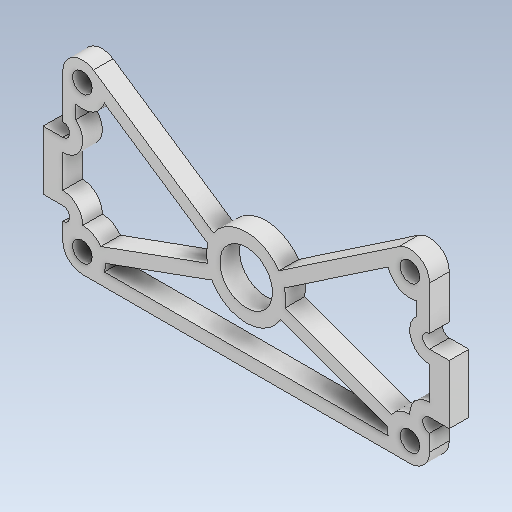
# Autodesk Inventor part: 横回転フレーム改３
Saved by Autodesk Inventor 2020 (Build 240168000, 168)
## iProperties
Created: 2020-02-25
Part Number: 横回転フレーム改３
Material: アルミニウム 2014-T4
Document SubType Name: Modeling
Designer: tanjihayato
Density: 2.8 g/cm^3
Appearance: サテン
Mass: 4.28179 g
Surface Area: 24.5942 cm^2
Volume: 1.52921 cm^3
Author: tanjihayato
Autodesk Inventor part; units mm, degrees
ref_plane "YZ Plane" through (0, 0, 0) normal (1, 0, 0) x (0, 1, 0)
ref_plane "XZ Plane" through (0, 0, 0) normal (0, 1, 0) x (-1, 0, 0)
ref_plane "XY Plane" through (0, 0, 0) normal (0, 0, 1) x (1, 0, 0)
sketch "スケッチ1" plane through (0, 0, 0) normal (0, 0, 1) x (1, 0, 0)
  line L0 (0, 0) -> (0, 4) construction
  line L1 (0, 0) -> (8.6476, -12.2564)
  line L2 (8.6476, -12.2564) -> (-0.2755, 4.5179)
  circle A0 centre (3.0119, -1.6621) radius 4
  line L3 (-57.3278, -140) -> (69.8706, -140)
  line L4 (3.0119, -1.6621) -> (117.7837, 59.3906)
  circle A1 centre (0, 0) radius 23.1
  circle A2 centre (0, -29.1039) radius 6.0039
  line L5 (0, 0) -> (0, -29.1039) construction
  circle A3 centre (0, -29.1039) radius 16.55
  circle A4 centre (0, -7.5039) radius 5.05
  circle A5 centre (0, 4) radius 3
  circle A6 centre (0, -7.5039) radius 20.05
  circle A7 centre (-14, 10.2376) radius 2.55
  circle A8 centre (14, 10.2376) radius 2.55
  circle A9 centre (14, -25.2454) radius 2.55
  circle A10 centre (-14, -25.2454) radius 2.55
  circle A11 centre (-14, 10.2376) radius 14
  circle A12 centre (14, 10.2376) radius 14
  circle A13 centre (14, -25.2454) radius 14
  circle A14 centre (-14, -25.2454) radius 14
  line L6 (-14, 10.2376) -> (-14, -25.2454) construction
  line L7 (-14, -25.2454) -> (14, -25.2454) construction
  circle A15 centre (0, 0) radius 9
  line L8 (-0.2755, 4.5179) -> (3.4816, -2.5449) construction
  line L9 (-2.9462, 3.0973) -> (0.8109, -3.9656)
  line L10 (6.1522, -1.1243) -> (2.3951, 5.9386)
  arc A16 (2.3951, 5.9386) -> (-2.9462, 3.0973) centre (-0.2755, 4.5179) ccw
  arc A17 (0.8109, -3.9656) -> (6.1522, -1.1243) centre (3.4816, -2.5449) ccw
  line L11 (-5, 2.8868) -> (5, 2.8868) construction
  line L12 (5, 2.8868) -> (0, -5.7735) construction
  line L13 (0, -5.7735) -> (-5, 2.8868) construction
  circle A18 centre (-5, 2.8868) radius 1.5
  circle A19 centre (5, 2.8868) radius 1.5
  circle A20 centre (0, -5.7735) radius 1.5
  line L14 (-28, 22.5965) -> (-28, -43.3295)
  line L15 (28, 22.9271) -> (28, -43.0008)
  line L16 (-28, 26.1991) -> (28, 26.1991)
  circle A21 centre (0, 0) radius 25.1
  line L17 (-28, -18.848) -> (28, -18.848)
  circle A22 centre (0, -29.1039) radius 8.0039
  circle A23 centre (-25, 23.1991) radius 3
  circle A24 centre (25, 23.1991) radius 3
  circle A25 centre (25, -38.2069) radius 3
  circle A26 centre (-25, -38.2069) radius 3
  circle A27 centre (-25, -15.848) radius 3
  circle A28 centre (25, -15.848) radius 3
  circle A29 centre (-25, -15.848) radius 4.5
  circle A30 centre (25, -15.848) radius 4.5
  circle A31 centre (0, -7.5039) radius 4.5
  circle A32 centre (0, -29.1039) radius 17.55
  circle A33 centre (0, -7.5039) radius 6.05
  point P0 (1.603, 0.9865)
  dimension "d0" = 4
  dimension "d1" = 15
  dimension "d2" = 18.4133
  dimension "d3" = 19
  dimension "d4" = 8
  dimension "d5" = 12
  dimension "d6" = 140
  dimension "d7" = 130
  dimension "d8" = 46.2
  dimension "d9" = 29.1039
  dimension "d10" = 33.1
  dimension "d11" = 10.1
  dimension "d12" = 6
  dimension "d13" = 40.1
  dimension "d14" = 28
  dimension "d15" = 28
  dimension "d16" = 28
  dimension "d17" = 28
  dimension "d18" = 18
  dimension "d19" = 8
  dimension "d20" = 6.05
  dimension "d21" = 3
  dimension "d22" = 3
  dimension "d23" = 3
  dimension "d24" = 10
  dimension "d25" = 2
  dimension "d26" = 2
  dimension "d27" = 6
  dimension "d28" = 6
  dimension "d29" = 6
  dimension "d30" = 6
  dimension "d31" = 6
  dimension "d32" = 6
  dimension "d33" = 9
  dimension "d34" = 9
  dimension "d35" = 9
  dimension "d36" = 5.1
  dimension "d37" = 1
  dimension "d38" = 1
  dimension "d39" = 56
  dimension "d40" = 28
  constraints: 38 end point, 34 centre point, 26 tangent, 16 coincident, 8 point on line, 5 vertical, 4 point on circle, 3 equal radius, 3 horizontal, 3 perpendicular, 1 midpoint, 1 parallel, 7 other
  measures "d0" distance of L0.start L0.end
  measures "d1" distance of L0.start L1.end
  measures "d2" distance of L0.end L1.end
  measures "d3" distance of L1.end L2.end
  measures "d4" diameter of A0
  measures "d5" distance of L1.end L4.start
  measures "d6" distance from line of L3 L0.start
  measures "d7" distance of L4.start L4.end
  measures "d8" diameter of A1
  measures "d9" distance of L5.end L0.start
  measures "d10" diameter of A3
  measures "d11" diameter of A4
  measures "d12" diameter of A5
  measures "d13" diameter of A6
  measures "d14" diameter of A11
  measures "d15" diameter of A12
  measures "d16" diameter of A13
  measures "d17" diameter of A14
  measures "d18" diameter of A15
  measures "d19" distance of L2.end L8.end
  measures "d20" diameter of A17
  measures "d21" diameter of A18
  measures "d22" diameter of A19
  measures "d23" diameter of A20
  measures "d24" distance of L11.end L12.end
  measures "d25" radial gap between concentric circles of A1 A21
  measures "d26" radial gap between concentric circles of A2 A22
  measures "d27" diameter of A23
  measures "d28" diameter of A24
  measures "d29" diameter of A25
  measures "d30" diameter of A26
  measures "d31" diameter of A27
  measures "d32" diameter of A28
  measures "d33" diameter of A29
  measures "d34" diameter of A30
  measures "d35" diameter of A31
  measures "d36" diameter of A7
  measures "d37" radial gap between concentric circles of A3 A32
  measures "d38" radial gap between concentric circles of A4 A33
  measures "d39" distance between parallel lines of L15 L14
  measures "d40" distance from line of A6.centre L15
sketch "スケッチ2" plane through (0, 0, 0) normal (0, 0, 1) x (1, 0, 0)
  circle A0 centre (-25, -15.848) radius 3 projected
  circle A1 centre (-25, -38.2069) radius 3 projected
  circle A2 centre (25, -38.2069) radius 3 projected
  circle A3 centre (25, -15.848) radius 3 projected
  circle A4 centre (0, -29.1039) radius 6.0039 construction
  circle A5 centre (0, 0) radius 25.1 construction
  circle A6 centre (0, -29.1039) radius 4.025
  line L0 (25, -41.2069) -> (-25, -41.2069)
  circle A7 centre (-25, -15.848) radius 1.5
  circle A8 centre (25, -15.848) radius 1.5
  circle A9 centre (25, -38.2069) radius 1.5
  circle A10 centre (-25, -38.2069) radius 1.5
  circle A11 centre (0, -29.1039) radius 6.025
  line L1 (23.3216, -13.3615) -> (4.9938, -25.733)
  line L2 (-4.9938, -25.733) -> (-23.3216, -13.3615)
  line L3 (-28, -15.848) -> (-28, -38.2069)
  line L4 (28, -15.848) -> (28, -38.2069)
  line L5 (-28, -24.6039) -> (-31, -24.6039)
  line L6 (-31, -24.6039) -> (-31, -33.6039)
  line L7 (-31, -33.6039) -> (-28, -33.6039)
  line L8 (28, -24.6039) -> (31, -24.6039)
  line L9 (31, -24.6039) -> (31, -33.6039)
  line L10 (31, -33.6039) -> (28, -33.6039)
  circle A12 centre (-28, -34.6539) radius 1.05
  circle A13 centre (-28, -23.5539) radius 1.05
  circle A14 centre (28, -23.5539) radius 1.05
  circle A15 centre (28, -34.6539) radius 1.05
  point P0 (-28, -22.5039)
  point P1 (-28, -35.7039)
  point P2 (28, -35.7039)
  point P3 (28, -22.5039)
  dimension "d41" = 8.05
  dimension "d52" = 3
  dimension "d53" = 3
  dimension "d54" = 3
  dimension "d55" = 3
  dimension "d57" = 2
  dimension "d61" = 3
  dimension "d62" = 9
  dimension "d63" = 3
  dimension "d64" = 9
  dimension "d65" = 2.1
  dimension "d66" = 2.1
  dimension "d67" = 2.1
  dimension "d68" = 2.1
  dimension "d69" = 4.5
  constraints: 22 end point, 12 point on line, 10 centre point, 10 point on circle, 9 tangent, 5 coincident, 3 perpendicular, 2 horizontal, 2 vertical, 1 parallel
  measures "d41" diameter of A6
  measures "d52" diameter of A7
  measures "d53" diameter of A8
  measures "d54" diameter of A9
  measures "d55" diameter of A10
  measures "d57" radial gap between concentric circles of A6 A11
  measures "d61" distance of L5.start L5.end
  measures "d62" distance of L5.end L6.end
  measures "d63" distance of L8.start L8.end
  measures "d64" distance of L8.end L9.end
  measures "d65" diameter of A12
  measures "d66" diameter of A13
  measures "d67" diameter of A14
  measures "d68" diameter of A15
  measures "d69" distance from line of L10 A4.centre
extrude "押し出し2" add sketch "スケッチ2" along normal blind 3 contours A0 | A0 L2 A11 L1 A3 L4 A14 A15 A2 L0 A1 L3 A12 A13 | A11 | L3 L7 L6 L5 | A3 | A1 | L8 L9 L10 L4 | A2
sketch "スケッチ3" plane through (0, 0, 3) normal (0, 0, 1) x (1, 0, 0)
  line L0 (-28, -15.848) -> (-28, -22.5039) projected
  arc A0 (-28, -24.6039) -> (-28, -22.5039) centre (-28, -23.5539) ccw projected
  line L1 (-28, -24.6039) -> (-31, -24.6039) projected
  line L2 (-31, -24.6039) -> (-31, -33.6039) projected
  line L3 (-31, -33.6039) -> (-28, -33.6039) projected
  arc A1 (-28, -35.7039) -> (-28, -33.6039) centre (-28, -34.6539) ccw projected
  line L4 (-28, -35.7039) -> (-28, -38.2069) projected
  arc A2 (-28, -38.2069) -> (-25, -41.2069) centre (-25, -38.2069) ccw projected
  line L5 (-25, -41.2069) -> (25, -41.2069) projected
  arc A3 (25, -41.2069) -> (28, -38.2069) centre (25, -38.2069) ccw projected
  line L6 (28, -38.2069) -> (28, -35.7039) projected
  arc A4 (28, -33.6039) -> (28, -35.7039) centre (28, -34.6539) ccw projected
  line L7 (28, -33.6039) -> (31, -33.6039) projected
  line L8 (31, -33.6039) -> (31, -24.6039) projected
  line L9 (31, -24.6039) -> (28, -24.6039) projected
  arc A5 (28, -22.5039) -> (28, -24.6039) centre (28, -23.5539) ccw projected
  line L10 (28, -22.5039) -> (28, -15.848) projected
  arc A6 (28, -15.848) -> (23.3216, -13.3615) centre (25, -15.848) ccw projected
  line L11 (23.3216, -13.3615) -> (4.9938, -25.733) projected
  arc A7 (4.9938, -25.733) -> (-4.9938, -25.733) centre (0, -29.1039) ccw projected
  line L12 (-4.9938, -25.733) -> (-23.3216, -13.3615) projected
  arc A8 (-23.3216, -13.3615) -> (-28, -15.848) centre (-25, -15.848) ccw projected
  circle A9 centre (25, -38.2069) radius 1.5 projected
  circle A10 centre (-25, -38.2069) radius 1.5 projected
  circle A11 centre (25, -15.848) radius 1.5 projected
  circle A12 centre (0, -29.1039) radius 4.025 projected
  circle A13 centre (-25, -15.848) radius 1.5 projected
  line L13 (-24.4405, -15.0192) -> (-4.0141, -28.8074)
  arc A14 (4.0141, -28.8074) -> (-4.0141, -28.8074) centre (0, -29.1039) ccw
  line L14 (4.0141, -28.8074) -> (24.4405, -15.0192)
  arc A15 (26, -15.848) -> (24.4405, -15.0192) centre (25, -15.848) ccw
  line L15 (26, -15.848) -> (26, -21.2512)
  arc A16 (26, -21.2512) -> (28, -26.6039) centre (28, -23.5539) ccw
  line L16 (28, -26.6039) -> (29, -26.6039)
  line L17 (29, -26.6039) -> (29, -31.6039)
  line L18 (29, -31.6039) -> (28, -31.6039)
  arc A17 (28, -31.6039) -> (26, -36.9566) centre (28, -34.6539) ccw
  line L19 (26, -36.9566) -> (26, -38.2069)
  arc A18 (25, -39.2069) -> (26, -38.2069) centre (25, -38.2069) ccw
  line L20 (25, -39.2069) -> (-25, -39.2069)
  arc A19 (-26, -38.2069) -> (-25, -39.2069) centre (-25, -38.2069) ccw
  line L21 (-26, -38.2069) -> (-26, -36.9566)
  arc A20 (-26, -36.9566) -> (-28, -31.6039) centre (-28, -34.6539) ccw
  line L22 (-28, -31.6039) -> (-29, -31.6039)
  line L23 (-29, -31.6039) -> (-29, -26.6039)
  line L24 (-29, -26.6039) -> (-28, -26.6039)
  arc A21 (-28, -26.6039) -> (-26, -21.2512) centre (-28, -23.5539) ccw
  line L25 (-26, -21.2512) -> (-26, -15.848)
  arc A22 (-24.4405, -15.0192) -> (-26, -15.848) centre (-25, -15.848) ccw
  circle A23 centre (0, -29.1039) radius 6.025
  circle A24 centre (25, -15.848) radius 3.5
  circle A25 centre (25, -38.2069) radius 3.5
  circle A26 centre (-25, -38.2069) radius 3.5
  circle A27 centre (-25, -15.848) radius 3.5
  line L26 (-25, -38.2069) -> (0, -29.1039) construction
  line L27 (-24.6579, -39.1465) -> (0.3421, -30.0435)
  line L28 (-0.3421, -28.1643) -> (-25.3421, -37.2672)
  arc A28 (-25.3421, -37.2672) -> (-24.6579, -39.1465) centre (-25, -38.2069) ccw
  arc A29 (0.3421, -30.0435) -> (-0.3421, -28.1643) centre (0, -29.1039) ccw
  line L29 (0, -29.1039) -> (25, -38.2069) construction
  line L30 (-0.3421, -30.0435) -> (24.6579, -39.1465)
  line L31 (25.3421, -37.2672) -> (0.3421, -28.1643)
  arc A30 (0.3421, -28.1643) -> (-0.3421, -30.0435) centre (0, -29.1039) ccw
  arc A31 (24.6579, -39.1465) -> (25.3421, -37.2672) centre (25, -38.2069) ccw
  line L32 (-28, -22.5039) -> (-28, -35.7039)
  line L33 (28, -38.2069) -> (28, -35.7039) projected
  line L34 (28, -22.5039) -> (28, -35.7039)
  point P0 (0, 0)
  point P1 (-12.5, -33.6554)
  point P2 (12.5, -33.6554)
  point P3 (28, -26.6039)
  point P4 (26, -19.2021)
  point P5 (21.6605, -16.8957)
  point P6 (5.8296, -27.5818)
  point P7 (5.925, -30.1971)
  point P8 (22.1905, -36.1196)
  point P9 (24.9505, -34.7072)
  point P10 (21.5062, -37.9989)
  point P11 (5.2407, -32.0764)
  point P12 (-5.2407, -32.0764)
  point P13 (-21.5062, -37.9989)
  point P14 (-21.6459, -39.2069)
  point P15 (21.6459, -39.2069)
  point P16 (-28, -31.6039)
  point P17 (-24.9505, -34.7072)
  point P18 (-22.1905, -36.1196)
  point P19 (-5.925, -30.1971)
  point P20 (-5.8296, -27.5818)
  point P21 (-21.6605, -16.8957)
  point P22 (-26, -19.2021)
  dimension "d72" = 2
  dimension "d73" = 2
  dimension "d74" = 2
  dimension "d75" = 2
  dimension "d76" = 2
  dimension "d77" = 2
  dimension "d78" = 2
  dimension "d79" = 2
  constraints: 46 end point, 26 point on circle, 18 centre point, 8 tangent, 3 parallel, 2 midpoint, 1 vertical, 21 other
  measures "d72" distance between parallel lines of L12 L13
  measures "d73" radial gap between concentric circles of A12 A23
  measures "d74" radial gap between concentric circles of A11 A24
  measures "d75" radial gap between concentric circles of A9 A25
  measures "d76" radial gap between concentric circles of A10 A26
  measures "d77" radial gap between concentric circles of A13 A27
  measures "d78" diameter of A29
  measures "d79" diameter of A31
extrude "押し出し3" cut sketch "スケッチ3" against normal blind 10 contours A27 L13 A23 L28 A26 A20 L32 A21 L25 | L14 A24 L15 A16 L34 A17 A25 L31 A23 | A23 L30 A25 L20 A26 L27
equation "\"d14\" = d15"
equation "\"d16\" = d15"
equation "\"d17\" = d14"
equation "\"d40\" = 0.5 * d39"
